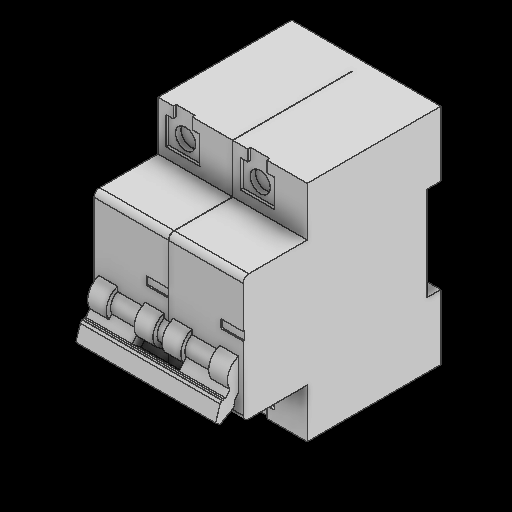
# Autodesk Inventor part: Breaker
Saved by Autodesk Inventor 2025.2 (Build 292293000, 293)
## iProperties
Created: 2026-05-14
Part Number: Breaker
Material: Generic
Document SubType Name: Modeling
Designer: valer
Density: 1 g/cm^3
Appearance: Default
Author: valer
Autodesk Inventor part; units mm, degrees
ref_plane "YZ Plane" through (0, 0, 0) normal (1, 0, 0) x (0, 1, 0)
ref_plane "XZ Plane" through (0, 0, 0) normal (0, 1, 0) x (-1, 0, 0)
ref_plane "XY Plane" through (0, 0, 0) normal (0, 0, 1) x (1, 0, 0)
sketch "Base" plane through (0, 0, 0) normal (0, 0, 1) x (1, 0, 0)
  line L0 (-26.8, -40.2) -> (26.8, -40.2)
  line L1 (26.8, -40.2) -> (26.8, 40.2)
  line L2 (26.8, 40.2) -> (-26.8, 40.2)
  line L3 (-26.8, 40.2) -> (-26.8, -40.2)
  line L4 (-26.8, -40.2) -> (26.8, 40.2) construction
  line L5 (26.8, -40.2) -> (-26.8, 40.2) construction
  point P0 (0, 0)
  dimension "d0" = 80.4
  dimension "d1" = 53.6
  constraints: 12 end point, 2 midpoint, 2 parallel, 1 horizontal, 1 perpendicular
  measures "d0" distance of L2.end L0.start
  measures "d1" distance of L0.start L0.end
extrude "BaseFeature" add sketch "Base" along normal blind 48
sketch "DINRail" plane through (-26.8, -40.2, 0) normal (-1, 0, 0) x (0, 0, 1)
  line L0 (0, 80.4) -> (0, 0) construction
  line L1 (0, 0) -> (48, 0) construction
  line L2 (48, 80.4) -> (48, 0) construction
  line L3 (0, 80.4) -> (48, 80.4) construction
  line L4 (0, 57.05) -> (5, 57.05)
  line L5 (5, 57.05) -> (5, 23.35)
  line L6 (5, 23.35) -> (0, 23.35)
  line L7 (0, 23.35) -> (0, 57.05)
  line L8 (0, 57.05) -> (5, 23.35) construction
  line L9 (5, 57.05) -> (0, 23.35) construction
  line L10 (0, -16.08) -> (0, 96.48) projected
  line L11 (-9.6, 40.2) -> (57.6, 40.2) construction
  line L12 (0, 80.4) -> (0, 0) projected
  point P0 (2.5, 40.2)
  point P1 (0, -16.08)
  dimension "d4" = 5
  dimension "d5" = 33.7
  constraints: 12 end point, 2 midpoint, 2 parallel, 1 horizontal, 1 perpendicular, 1 point on line, 1 vertical, 2 other
  measures "d4" distance of L4.start L4.end
  measures "d5" distance of L6.end L4.start
extrude "DinRailFeature" cut sketch "DINRail" against normal through all
sketch "Top" plane through (0, 0, 48) normal (0, 0, 1) x (1, 0, 0)
  line L0 (26.8, -40.2) -> (26.8, 40.2) projected
  line L1 (-26.8, -22.575) -> (26.8, -22.575)
  line L2 (26.8, -22.575) -> (26.8, 22.575)
  line L3 (26.8, 22.575) -> (-26.8, 22.575)
  line L4 (-26.8, 22.575) -> (-26.8, -22.575)
  line L5 (-26.8, -22.575) -> (26.8, 22.575) construction
  line L6 (26.8, -22.575) -> (-26.8, 22.575) construction
  point P0 (0, 0)
  point P1 (26.8, -22.575)
  dimension "d31" = 45.15
  constraints: 12 end point, 2 midpoint, 2 parallel, 1 horizontal, 1 perpendicular, 1 point on line
  measures "d31" distance between parallel lines of L1 L3
extrude "TopFeature" add sketch "Top" along normal blind 23
fillet "TopFilletsFeature" radius 2 2 edges at (0, 22.575, 71) (0, -22.575, 71)
sketch "PartingLine" plane through (0, 0, 71) normal (0, 0, 1) x (1, 0, 0)
  line L0 (26.8, 40.2) -> (-26.8, 40.2) projected
  line L1 (-26.8, -40.2) -> (26.8, -40.2) projected
  line L2 (-0.05, 40.2) -> (0.05, 40.2)
  line L3 (0.05, 40.2) -> (0.05, -40.2)
  line L4 (0.05, -40.2) -> (-0.05, -40.2)
  line L5 (-0.05, -40.2) -> (-0.05, 40.2)
  line L6 (0, -56.28) -> (0, 56.28) construction
  point P0 (0, 0)
  point P1 (0, 40.2)
  dimension "d71" = 0.1
  constraints: 8 end point, 3 point on line, 2 parallel, 1 horizontal, 1 midpoint, 1 perpendicular
  measures "d71" distance between parallel lines of L3 L5
sketch "SwitchHood" plane through (26.8, -40.2, 48) normal (1, 0, 0) x (0, 0, -1)
  line L0 (-23, 60.775) -> (-23, 19.625) projected
  circle A0 centre (-21, 31.625) radius 6
  line L1 (-21, 31.625) -> (-27, 31.625) construction
  line L2 (-21, 31.625) -> (-21, 25.625) construction
  line L3 (0, 17.625) -> (-21, 17.625) projected
  point P0 (48, 40.2)
  point P1 (-23, 25.9681)
  point P2 (-23, 37.2819)
  dimension "d35" = 12
  dimension "d36" = 4
  dimension "d37" = 8
  constraints: 4 end point, 2 point on circle, 1 centre point, 1 horizontal, 1 vertical
  measures "d35" diameter of A0
  measures "d36" distance from line of L0 L1.end
  measures "d37" distance from line of L2.end L3
extrude "SwitchHoodFeature" add sketch "SwitchHood" against normal up to surface (53.6 mm away) contours L0 A0 picked at (-25.1519, 32.1124)
sketch "SwithCuts" plane through (0, 0, 71) normal (0, 0, 1) x (1, 0, 0)
  line L0 (26.8, -2.9181) -> (26.8, 20.575) projected
  line L1 (26.8, -14.2319) -> (-26.8, -14.2319) projected
  line L2 (26.8, -2.9181) -> (25.1, -2.9181)
  line L3 (25.1, -2.9181) -> (25.1, -14.2319)
  line L4 (25.1, -14.2319) -> (26.8, -14.2319)
  line L5 (26.8, -14.2319) -> (26.8, -2.9181)
  line L6 (0, 56.28) -> (0, -56.28) construction
  line L7 (-26.8, -2.9181) -> (-25.1, -2.9181)
  line L8 (-25.1, -2.9181) -> (-25.1, -14.2319)
  line L9 (-25.1, -14.2319) -> (-26.8, -14.2319)
  line L10 (-26.8, -14.2319) -> (-26.8, -2.9181)
  line L11 (-26.8, -2.9181) -> (26.8, -2.9181) projected
  line L12 (-1.65, -2.9181) -> (1.65, -2.9181)
  line L13 (1.65, -2.9181) -> (1.65, -14.2319)
  line L14 (1.65, -14.2319) -> (-1.65, -14.2319)
  line L15 (-1.65, -14.2319) -> (-1.65, -2.9181)
  line L16 (-25.1, -2.9181) -> (-1.65, -14.2319) construction
  line L17 (1.65, -2.9181) -> (25.1, -14.2319) construction
  line L18 (-18.375, -14.2319) -> (-8.375, -14.2319)
  line L19 (-8.375, -14.2319) -> (-8.375, -2.9181)
  line L20 (-8.375, -2.9181) -> (-18.375, -2.9181)
  line L21 (-18.375, -2.9181) -> (-18.375, -14.2319)
  line L22 (-18.375, -14.2319) -> (-8.375, -2.9181) construction
  line L23 (-8.375, -14.2319) -> (-18.375, -2.9181) construction
  line L24 (18.375, -14.2319) -> (8.375, -14.2319)
  line L25 (8.375, -14.2319) -> (8.375, -2.9181)
  line L26 (8.375, -2.9181) -> (18.375, -2.9181)
  line L27 (18.375, -2.9181) -> (18.375, -14.2319)
  point P0 (0, 0)
  point P1 (-13.375, -8.575)
  point P2 (8.375, -2.9181)
  point P3 (8.375, -14.2319)
  point P4 (18.375, -14.2319)
  point P5 (18.375, -2.9181)
  point P6 (-18.375, -2.9181)
  point P7 (-18.375, -14.2319)
  point P8 (-8.375, -14.2319)
  point P9 (-8.375, -2.9181)
  point P10 (-1.65, -14.2319)
  point P11 (1.65, -2.9181)
  point P12 (-26.8, -14.2319)
  point P13 (-25.1, -14.2319)
  point P14 (0, -2.9181)
  dimension "d40" = 1.7
  dimension "d43" = 10
  dimension "d74" = 3.3
  constraints: 48 end point, 8 symmetric about line, 6 parallel, 4 midpoint, 4 point on line, 3 horizontal, 3 perpendicular, 1 collinear
  measures "d40" distance between parallel lines of L5 L3
  measures "d43" distance of L19.end L20.end
  measures "d74" distance between parallel lines of L13 L15
extrude "SwitchCutsFeature" cut sketch "SwithCuts" along normal through all contours L1 L3 L2 L5 | L1 L25 L11 L27 | L1 L15 L11 L13 | L1 L21 L11 L19 | L1 L10 L7 L8
sketch "SwitchBase" plane through (-25.1, -14.2319, 71) normal (-1, 0, 0) x (0, 0, 1)
  arc A0 (0, 0) -> (0, 11.3137) centre (-2, 5.6569) ccw projected
  circle A1 centre (-2, 5.6569) radius 4.5
  point P0 (-71, 14.2319)
  dimension "d46" = 1.5
  constraints: 1 centre point, 1 coincident
  measures "d46" radial gap between concentric circles of A0 A1
extrude "SwitchBaseFeature" add sketch "SwitchBase" against normal up to surface (50.2 mm away)
sketch "Switch" plane through (-25.1, -14.2319, 71) normal (-1, 0, 0) x (0, 0, 1)
  arc A0 (0, 1.6257) -> (0, 9.688) centre (-2, 5.6569) ccw projected
  line L0 (-9.8725, 18.5806) -> (8.9836, -4.7527)
  line L1 (8.9836, -4.7527) -> (5.8725, -7.2669)
  line L2 (5.8725, -7.2669) -> (-12.9836, 16.0664)
  line L3 (-12.9836, 16.0664) -> (-9.8725, 18.5806)
  line L4 (-9.8725, 18.5806) -> (5.8725, -7.2669) construction
  line L5 (8.9836, -4.7527) -> (-12.9836, 16.0664) construction
  point P0 (-71, 14.2319)
  point P1 (-2, 5.6569)
  point P2 (0, 0)
  dimension "d49" = 4
  dimension "d50" = 15
  constraints: 12 end point, 3 midpoint, 2 parallel, 1 perpendicular, 1 point on line
  measures "d49" distance of L0.end L1.end
  measures "d50" distance from line of point (-2, 5.657) L1
extrude "SwitchFeature" add sketch "Switch" against normal up to surface (50.2 mm away)
sketch "SwitchTop" plane through (-25.1, -14.2319, 71) normal (-1, 0, 0) x (0, 0, 1)
  line L0 (3.1111, 2.5142) -> (8.9836, -4.7527) projected
  line L1 (4.6442, 0.6171) -> (5.287, 0.6171)
  line L2 (5.287, 0.6171) -> (5.6013, 0.2282)
  line L3 (5.6013, 0.2282) -> (5.9902, 0.5425)
  line L4 (5.9902, 0.5425) -> (6.6187, -0.2353)
  line L5 (6.6187, -0.2353) -> (8.2059, -5.3813)
  line L6 (5.8725, -7.2669) -> (8.9836, -4.7527) projected
  arc A0 (3.1111, 2.5142) -> (0, 11.3137) centre (-2, 5.6569) ccw projected
  line L7 (7.4281, -6.0098) -> (-2, 5.6569) construction
  line L8 (1.5331, -1.8971) -> (1.3981, -2.5256)
  line L9 (1.3981, -2.5256) -> (1.7124, -2.9145)
  line L10 (1.7124, -2.9145) -> (1.3235, -3.2288)
  line L11 (1.3235, -3.2288) -> (1.9521, -4.0065)
  line L12 (1.9521, -4.0065) -> (6.6503, -6.6384)
  line L13 (0, 0) -> (5.8725, -7.2669) projected
  point P0 (-71, 14.2319)
  point P1 (4.3012, -5.3224)
  point P2 (7.4123, -2.8083)
  point P3 (6.6503, -6.6384)
  dimension "d53" = 6
  dimension "d54" = 1
  dimension "d55" = 0.5
  dimension "d56" = 0.5
  dimension "d57" = 0.5
  dimension "d58" = 1
  constraints: 22 end point, 6 symmetric about line, 2 perpendicular, 2 point on line, 1 horizontal, 1 midpoint, 1 parallel
  measures "d53" distance between parallel lines of L6 L3
  measures "d54" distance of L3.end L4.end
  measures "d55" distance of L2.end L3.end
  measures "d56" distance between parallel lines of L0 L2
  measures "d57" distance of L1.end L2.end
  measures "d58" distance of L5.end L0.end
extrude "SwitchOutside" add sketch "SwitchTop" against normal up to surface (50.2 mm away) contours L1 L2 L3 L4 L5 L0 | L0 L6 L5 | L12 L11 L10 L9 L8 L13
extrude "SwitchTopFeature" cut sketch "SwitchTop" against normal through all contours L0 L6 L5 | L13 L12 L6
sketch "SwitchInside" plane through (8.375, -10.4532, 73.0893) normal (0, 0.6285394, 0.7777778) x (1, 0, 0)
  line L0 (-33.475, -4.0648) -> (16.725, -4.0648) projected
  line L1 (16.725, -1.6257) -> (16.725, -4.0648) projected
  line L2 (10, 0) -> (10, -1.6257) projected
  line L3 (0, 0) -> (10, 0) projected
  line L4 (0, -1.6257) -> (0, 0) projected
  line L5 (-6.725, -1.6257) -> (0, -1.6257) projected
  line L6 (-6.725, 0) -> (-6.725, -1.6257) projected
  line L7 (-10.025, 0) -> (-6.725, 0) projected
  line L8 (-10.025, -1.6257) -> (-10.025, 0) projected
  line L9 (-16.75, -1.6257) -> (-10.025, -1.6257) projected
  line L10 (-16.75, 0) -> (-16.75, -1.6257) projected
  line L11 (-26.75, 0) -> (-16.75, 0) projected
  line L12 (-26.75, -1.6257) -> (-26.75, 0) projected
  line L13 (-33.475, -4.0648) -> (-33.475, -1.6257) projected
  line L14 (-16.75, -1.6257) -> (-16.75, -4.0648)
  line L15 (-33.475, -4.0648) -> (16.725, -4.0648) projected
  line L16 (0, -1.6257) -> (0, -4.0648)
  line L17 (10, -1.6257) -> (16.725, -1.6257) projected
  line L18 (-33.475, -1.6257) -> (-26.75, -1.6257) projected
  point P0 (-8.375, 54.0698)
  constraints: 4 end point, 2 perpendicular, 2 point on line
extrude "SwitchInsideFeature" cut sketch "SwitchInside" against normal up to surface (4 mm away) contours L14 L9 L8 L7 L6 L5 L16 L0
extrude "PartingLineFeature" cut sketch "PartingLine" against normal up to surface (66 mm away)
sketch "TerminalIndents" plane through (0, 0, 48) normal (0, 0, 1) x (1, 0, 0)
  line L0 (-0.05, 22.575) -> (-0.05, 40.2) projected
  line L1 (-0.05, 40.2) -> (-26.8, 40.2) projected
  line L2 (-26.8, 40.2) -> (-26.8, 22.575) projected
  line L3 (-26.8, 22.575) -> (-0.05, 22.575) projected
  line L4 (0.05, 40.2) -> (0.05, 22.575) projected
  line L5 (0.05, 22.575) -> (26.8, 22.575) projected
  line L6 (26.8, 22.575) -> (26.8, 40.2) projected
  line L7 (26.8, 40.2) -> (0.05, 40.2) projected
  line L8 (-0.05, -40.2) -> (-0.05, -22.575) projected
  line L9 (-0.05, -22.575) -> (-26.8, -22.575) projected
  line L10 (-26.8, -22.575) -> (-26.8, -40.2) projected
  line L11 (-26.8, -40.2) -> (-0.05, -40.2) projected
  line L12 (0.05, -22.575) -> (0.05, -40.2) projected
  line L13 (0.05, -40.2) -> (26.8, -40.2) projected
  line L14 (26.8, -40.2) -> (26.8, -22.575) projected
  line L15 (26.8, -22.575) -> (0.05, -22.575) projected
  line L16 (-21.3, 40.2) -> (-14.5, 40.2)
  line L17 (-14.5, 40.2) -> (-14.5, 36.2)
  line L18 (-14.5, 36.2) -> (-21.3, 36.2)
  line L19 (-21.3, 36.2) -> (-21.3, 40.2)
  line L20 (-23.975, 36.2) -> (-11.825, 36.2)
  line L21 (-11.825, 36.2) -> (-11.825, 26.2)
  line L22 (-11.825, 26.2) -> (-23.975, 26.2)
  line L23 (-23.975, 26.2) -> (-23.975, 36.2)
  line L24 (26.8, 40.2) -> (-26.8, 40.2) projected
  line L25 (5.5, 40.2) -> (12.3, 40.2)
  line L26 (12.3, 40.2) -> (12.3, 36.2)
  line L27 (12.3, 36.2) -> (5.5, 36.2)
  line L28 (5.5, 36.2) -> (5.5, 40.2)
  line L29 (2.825, 36.2) -> (14.975, 36.2)
  line L30 (14.975, 36.2) -> (14.975, 26.2)
  line L31 (14.975, 26.2) -> (2.825, 26.2)
  line L32 (2.825, 26.2) -> (2.825, 36.2)
  line L33 (0, -56.28) -> (0, 56.28) construction
  line L34 (-37.52, 0) -> (37.52, 0) construction
  line L35 (-14.5, -40.2) -> (-14.5, -36.2)
  line L36 (-21.3, -36.2) -> (-21.3, -40.2)
  line L37 (-23.975, -36.2) -> (-11.825, -36.2)
  line L38 (-11.825, -36.2) -> (-11.825, -26.2)
  line L39 (-11.825, -26.2) -> (-23.975, -26.2)
  line L40 (-23.975, -26.2) -> (-23.975, -36.2)
  line L41 (12.3, -40.2) -> (12.3, -36.2)
  line L42 (5.5, -36.2) -> (5.5, -40.2)
  line L43 (2.825, -36.2) -> (14.975, -36.2)
  line L44 (14.975, -36.2) -> (14.975, -26.2)
  line L45 (14.975, -26.2) -> (2.825, -26.2)
  line L46 (2.825, -26.2) -> (2.825, -36.2)
  point P0 (0, 0)
  point P1 (-17.9, 36.2)
  point P2 (8.9, 36.2)
  dimension "d75" = 5.5
  dimension "d76" = 6.8
  dimension "d77" = 12.15
  dimension "d78" = 10
  dimension "d79" = 4
  dimension "d80" = 5.5
  constraints: 56 end point, 16 symmetric about line, 8 parallel, 4 equal length, 4 horizontal, 4 midpoint, 4 perpendicular, 2 point on line
  measures "d75" distance between parallel lines of L19 L2
  measures "d76" distance of L17.end L18.end
  measures "d77" distance of L21.end L22.end
  measures "d78" distance of L22.end L20.start
  measures "d79" distance of L16.end L17.end
  measures "d80" distance between parallel lines of L28 L33
extrude "TerminalIndentsFeature" cut sketch "TerminalIndents" against normal blind 1 contours L17 L18 L19 L1 | L20 L21 L22 L23 L18 | L7 L26 L27 L28 | L27 L29 L30 L31 L32 | L11 L36 L37 L35 | L37 L40 L39 L38 | L42 L43 L41 L13 | L43 L46 L45 L44
sketch "TerminalScrews" plane through (0, 0, 47) normal (0, 0, 1) x (1, 0, 0)
  line L0 (-23.975, 36.2) -> (-21.3, 36.2) construction
  line L1 (-11.825, 26.2) -> (-23.975, 26.2) construction
  line L2 (-23.975, 36.2) -> (-11.825, 26.2) construction
  line L3 (2.825, 36.2) -> (5.5, 36.2) construction
  line L4 (14.975, 26.2) -> (2.825, 26.2) construction
  line L5 (2.825, 36.2) -> (14.975, 26.2) construction
  line L6 (-37.52, 0) -> (37.52, 0) construction
  circle A0 centre (-17.9, 31.2) radius 3.65
  circle A1 centre (8.9, 31.2) radius 3.65
  circle A2 centre (-17.9, -31.2) radius 3.65
  circle A3 centre (8.9, -31.2) radius 3.65
  point P0 (0, 0)
  dimension "d83" = 7.3
  constraints: 4 centre point, 4 end point, 2 midpoint, 2 symmetric about line, 1 equal radius, 2 other
  measures "d83" diameter of A0
extrude "TerminalScrewsFeature" cut sketch "TerminalScrews" against normal blind 2
sketch "Viewports" plane through (0, 0, 71) normal (0, 0, 1) x (1, 0, 0)
  line L0 (26.8, -16.85) -> (26.8, 16.85) projected
  line L1 (26.8, 2.575) -> (18.8, 2.575)
  line L2 (18.8, 2.575) -> (18.8, 5.575)
  line L3 (18.8, 5.575) -> (26.8, 5.575)
  line L4 (26.8, 5.575) -> (26.8, 2.575)
  line L5 (-0.05, 16.85) -> (-0.05, -16.85) projected
  line L6 (-0.05, 2.575) -> (-8.05, 2.575)
  line L7 (-8.05, 2.575) -> (-8.05, 5.575)
  line L8 (-8.05, 5.575) -> (-0.05, 5.575)
  line L9 (-0.05, 5.575) -> (-0.05, 2.575)
  line L10 (26.8, 22.575) -> (0.05, 22.575) projected
  point P0 (0, 0)
  point P1 (-0.05, 5.575)
  dimension "d86" = 17
  dimension "d87" = 8
  dimension "d88" = 3
  constraints: 16 end point, 4 parallel, 3 collinear, 2 horizontal, 2 perpendicular, 2 point on line
  measures "d86" distance between parallel lines of L3 L10
  measures "d87" distance of L2.end L3.end
  measures "d88" distance of L1.end L2.end
extrude "ViewportsFeature" cut sketch "Viewports" against normal blind 0.5
equation "\"d80\" = d75"
body "Solid1"
